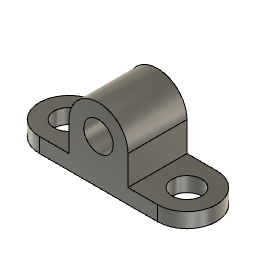
object A4 (Autodesk Fusion 360 design; units mm, degrees)
Autodesk Fusion 360 part; units mm, degrees
sketch "horizontal part sketch" plane through (0, 0, 0) normal (0, 0, 1) x (1, 0, 0)
  line L0 (-40, 20) -> (40, 20)
  line L1 (40, -20) -> (-40, -20)
  circle A0 centre (40, 0) radius 10
  circle A1 centre (-40, 0) radius 10
  arc A2 (-40, 20) -> (-40, -20) centre (-40, 0) ccw
  arc A3 (40, -20) -> (40, 20) centre (40, 0) ccw
  dimension "d1" = 40
  dimension "d2" = 80
  dimension "d5" = 40
  constraint horizontal L0
  constraint parallel L0 L1
  measures "d1" distance of L0.start L1.end
  measures "d2" distance of L0.start L0.end
  measures "d5" diameter of A3
extrude "Extrude1" add sketch "horizontal part sketch" along normal blind 10 makes body 1
sketch "vertical part sketch" plane through (0, 0, 0) normal (0, 1, 0) x (1, 0, 0)
  line L0 (-20, 0) -> (20, 0)
  line L1 (20, 0) -> (20, -30)
  line L2 (-20, -30) -> (-20, 0)
  line L3 (-40, 0) -> (-40, -10)
  circle A0 centre (0, -30) radius 10
  arc A1 (-20, -30) -> (20, -30) centre (0, -30) ccw
  dimension "d10" = 40
  dimension "d11" = 30
  dimension "d12" = 20
  dimension "d14" = 20
  constraint horizontal L0
  constraint vertical L1
  constraint vertical L2
  constraint concentric A0 A1
  measures "d10" distance of L0.start L0.end
  measures "d11" distance of L0.start L2.start
  measures "d12" distance of L2 L3
  measures "d14" diameter of A0
extrude "Extrude2" add sketch "vertical part sketch" along normal mid plane 40 bodies 1
copy_body "Body->Comp1" bodies 1 removing the originals makes body 2 in component "object A4"
component "object A4" placed x (1, 0, 0) y (0, 1, 0) z (0, 0, 1) at (0, 0, 0)
named bodies: "object A4"
